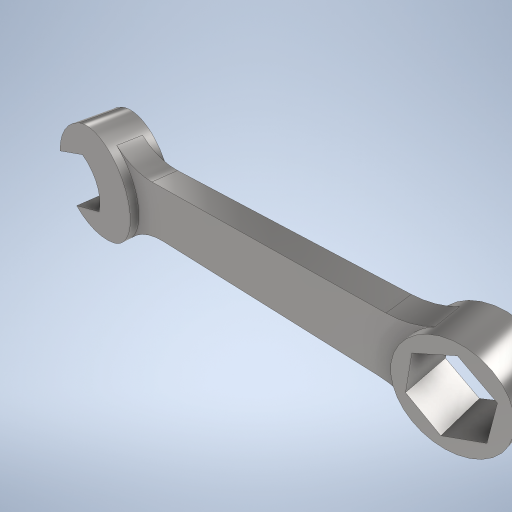
# Autodesk Inventor part: Co le
Saved by Autodesk Inventor 2024.3 (Build 283343000, 343)
## iProperties
Created: 2024-11-28
Part Number: Co le
Material: Steel, Alloy
Document SubType Name: Modeling
Designer: Admin
Density: 7.73 g/cm^3
Appearance: Semi-Polished
Author: Admin
Autodesk Inventor part; units mm, degrees
ref_plane "YZ Plane" through (0, 0, 0) normal (1, 0, 0) x (0, 1, 0)
ref_plane "XZ Plane" through (0, 0, 0) normal (0, 1, 0) x (-1, 0, 0)
ref_plane "XY Plane" through (0, 0, 0) normal (0, 0, 1) x (1, 0, 0)
sketch "Sketch1" plane through (0, 0, 0) normal (0, 0, 1) x (1, 0, 0)
  line L0 (0, 0) -> (0, 114.286) construction
  line L1 (0, 0) -> (-19.7038, 73.5356) construction
  ellipse E0 centre (0, 0) end of major axis (19.3185, 5.1764) minor radius 25 (6.4705, -24.1481) -> (-6.4705, 24.1481) ccw
  arc A0 (-1.3216, -12.7774) -> (-7.5332, 10.4048) centre (-17.3867, -4.6587) ccw
  line L2 (-7.5332, 10.4048) -> (-24.2902, 5.9148)
  line L3 (-1.3216, -12.7774) -> (-18.0786, -17.2675)
  arc A1 (-6.4705, 24.1481) -> (-24.2902, 5.9148) centre (0, 0) ccw
  arc A2 (-18.0786, -17.2675) -> (6.4705, -24.1481) centre (0, 0) ccw
  line L4 (0, 0) -> (160, 0) construction
  line L5 (30.4688, 12) -> (134.7611, 12)
  line L6 (34.1209, -12) -> (134.7611, -12)
  arc A3 (10.6834, 19.4492) -> (31.3482, 12.0129) centre (30.4688, 42) ccw
  arc A4 (34.1209, -12) -> (11.6572, -22.1158) centre (34.1209, -42) ccw
  circle A5 centre (160, 0) radius 19
  line L7 (172.9904, 7.5) -> (172.9904, -7.5)
  line L8 (172.9904, -7.5) -> (160, -15)
  line L9 (160, -15) -> (147.0096, -7.5)
  line L10 (147.0096, -7.5) -> (147.0096, 7.5)
  line L11 (147.0096, 7.5) -> (160, 15)
  line L12 (160, 15) -> (172.9904, 7.5)
  arc A6 (134.7611, 12) -> (150.2135, 16.2857) centre (134.7611, 42) ccw
  arc A7 (150.2135, -16.2857) -> (134.7611, -12) centre (134.7611, -42) ccw
  point P0 (172.9904, 0)
  point P1 (13.5706, -20.144)
  dimension "d12" = 20
  dimension "d14" = 25
  dimension "d19" = 38
  dimension "d7" = 15
  dimension "d10" = 18
  dimension "d13" = 24
  dimension "d15" = 25
  dimension "d16" = 30
  dimension "d17" = 24
  dimension "d18" = 30
  dimension "d20" = 30
  dimension "d21" = 160
  dimension "d23" = 15
  constraints: 26 end point, 17 point on circle, 7 centre point, 4 coincident, 4 tangent, 3 horizontal, 3 symmetric about line, 2 parallel, 2 point on line, 1 midpoint, 1 perpendicular, 1 vertical, 27 other
  measures "d7" angle of L0 L1
  measures "d10" radius of A0
  measures "d13" distance between parallel lines of L3 L2
  measures "d15" radius of A2
  measures "d16" radius of A3
  measures "d17" distance between parallel lines of L6 L5
  measures "d18" radius of A4
  measures "d20" radius of A6
  measures "d21" distance of L4.start L4.end
  measures "d23" distance of L7.end L8.end
extrude "Extrusion1" add sketch "Sketch1" along normal mid plane 20 contours E0 A2 L3 A0 L2 A1 | A5
extrude "Extrusion2" add sketch "Sketch1" along normal mid plane 12 contours A3 L5 A6 A5 A7 L6 A4 E0
body "Solid1"
